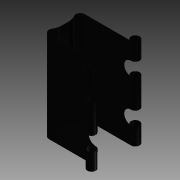
# Autodesk Inventor part: BINDER CLIP BODY
Saved by Autodesk Inventor 2013 (Build 170138000, 138)
## iProperties
Created: 2014-06-22
Part Number: BINDER CLIP BODY
Material: Generic
Document SubType Name: Modeling
Designer: employee
Density: 1 g/cm^3
Author: employee
Autodesk Inventor part; units mm, degrees
ref_plane "YZ Plane" through (0, 0, 0) normal (1, 0, 0) x (0, 1, 0)
ref_plane "XZ Plane" through (0, 0, 0) normal (0, 1, 0) x (-1, 0, 0)
ref_plane "XY Plane" through (0, 0, 0) normal (0, 0, 1) x (1, 0, 0)
sketch "Sketch1" plane through (0, 0, 0) normal (0, 0, 1) x (1, 0, 0)
  line L0 (0, 0) -> (0, 1.2859)
  arc A0 (0, 1.2859) -> (-0.7692, 3.9506) centre (-5, 1.2859) ccw
  arc A1 (0.5, 6.25) -> (-0.7692, 3.9506) centre (0.5, 4.75) ccw
  line L1 (0.5, 6.25) -> (17, 6.25)
  arc A2 (17, 6.25) -> (15.8298, 6.8115) centre (17, 7.75) ccw
  line L2 (0.5, 4.75) -> (-1, 4.75)
  dimension "d0" = 1.5
  dimension "d2" = 17
  dimension "d3" = 6.25
  dimension "d4" = 1
  dimension "d5" = 5
  constraints: 7 point on circle, 6 end point, 4 tangent, 3 centre point, 1 equal radius, 1 parallel, 1 perpendicular, 1 vertical
  measures "d0" radius of A2
  measures "d2" distance from line of A2.centre L0
  measures "d3" distance from line of L1 L0.start
  measures "d4" distance from line of L2.end L0
  measures "d5" radius of A0
sketch "Sketch2" plane through (0, 0, 0) normal (0, 1, 0) x (-1, 0, 0)
  line L0 (0.1, 16) -> (0, 16)
  line L1 (0, 16) -> (0, -16)
  line L2 (0, -16) -> (0.1, -16)
  line L3 (0.1, -16) -> (0.1, 16)
  point P0 (0, 0)
  point P1 (0, 0)
  dimension "d6" = 0.1
  dimension "d8" = 32
  constraints: 8 end point, 2 parallel, 1 coincident, 1 horizontal, 1 midpoint, 1 perpendicular
  measures "d6" distance of L0.start L0.end
  measures "d8" distance of L2.end L0.start
sweep "Sweep1" add profiles "Sketch2" path "Sketch1" path curves L0 A0 A1 L1 A2
sketch "Sketch3" plane through (0.5, 6.35, -16) normal (0, 1, 0) x (1, 0, 0)
  line L0 (0, 0) -> (16.5, 0) projected
  line L1 (0, -32) -> (0, 0) projected
  line L2 (0, -6) -> (24.5069, -6)
  line L3 (24.5069, -6) -> (24.5069, -11)
  line L4 (24.5069, -11) -> (0, -11)
  line L5 (0, -11) -> (0, -6)
  line L6 (0, -21) -> (24.5069, -21)
  line L7 (24.5069, -21) -> (24.5069, -26)
  line L8 (24.5069, -26) -> (0, -26)
  line L9 (0, -26) -> (0, -21)
  line L10 (24.5069, -21) -> (24.5069, -11)
  point P0 (-0.5, -16)
  point P1 (24.5069, -16)
  dimension "d10" = 5
  dimension "d12" = 6
  constraints: 18 end point, 4 parallel, 2 horizontal, 2 perpendicular, 2 point on line, 1 collinear, 1 horizontal alignment, 1 midpoint, 1 vertical
  measures "d10" distance of L2.end L3.end
  measures "d12" distance between parallel lines of L0 L2
extrude "Extrusion1" cut sketch "Sketch3" along normal through all contours L1 L6 L7 L8 | L1 L2 L3 L4
sketch "Sketch4" plane through (0.5, 6.35, -16) normal (0, 1, 0) x (1, 0, 0)
  line L0 (16.5, -26) -> (17.0385, -26) projected
  line L1 (16.5, -11) -> (17.0385, -11) projected
  circle A0 centre (16.5, -8.5) radius 2.5
  circle A1 centre (16.5, -23.5) radius 2.5
  point P0 (-0.5, -16)
  constraints: 2 centre point, 2 tangent, 2 vertical alignment
extrude "Extrusion2" cut sketch "Sketch4" along normal through all both and the other way through all
mirror "Mirror1" about plane through (-0.05, 0, 0) normal (0, -1, 0) of "Sweep1", "Extrusion1", "Extrusion2"
body "Solid1"
